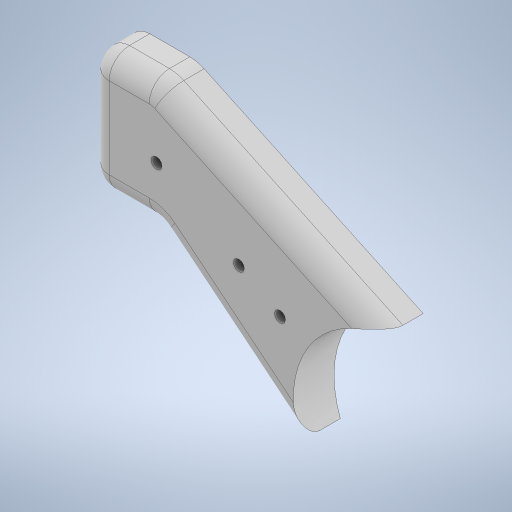
# Autodesk Inventor part: palec2
Saved by Autodesk Inventor 2024.2 (Build 282272000, 272)
## iProperties
Created: 2023-12-27
Part Number: palec2
Material: PLA
Document SubType Name: Modeling
Designer: Konrad
Density: 1 g/cm^3
Appearance: Domyślna
Author: Konrad
Autodesk Inventor part; units mm, degrees
ref_plane "YZ Plane" through (0, 0, 0) normal (1, 0, 0) x (0, 1, 0)
ref_plane "XZ Plane" through (0, 0, 0) normal (0, 1, 0) x (-1, 0, 0)
ref_plane "XY Plane" through (0, 0, 0) normal (0, 0, 1) x (1, 0, 0)
sketch "Szkic1" plane through (0, 0, 0) normal (0, 0, 1) x (1, 0, 0)
  circle A0 centre (0, 0) radius 4
  circle A1 centre (0, 0) radius 12.5 construction
  line L0 (0, 0) -> (-34.641, 20) construction
  line L1 (-44.641, 20) -> (-84.641, 20) construction
  line L2 (-34.641, 20) -> (-34.641, 30) construction
  line L3 (-34.641, 30) -> (5.2954, 11.3229)
  line L4 (-34.641, 20) -> (-34.641, 12) construction
  line L5 (-34.641, 12) -> (-7.8737, -9.7085)
  line L6 (-84.641, 20) -> (-84.641, 30)
  line L7 (-84.641, 30) -> (-34.641, 30)
  line L8 (-34.641, 12) -> (-39.641, 12)
  line L9 (-39.641, 12) -> (-39.641, 15) construction
  line L10 (-39.641, 20) -> (-34.641, 30) construction
  line L11 (-42.641, 20) -> (-37.641, 30) construction
  arc A2 (-1.3611, 14.436) -> (-13.5811, -5.0798) centre (0, 0) ccw
  line L12 (-104.0692, 0) -> (31.9282, 0) construction
  line L13 (-20.4848, 0.5192) -> (-10.0924, 18.5194) construction
  line L14 (-39.641, 12) -> (-44.641, 12)
  line L15 (-44.641, 12) -> (-44.641, 15)
  line L16 (-44.641, 15) -> (-39.641, 15) construction
  arc A3 (-39.641, 15) -> (-44.641, 20) centre (-44.641, 15) ccw
  arc A4 (-39.641, 15) -> (-36.641, 12) centre (-36.641, 15) ccw
  circle A5 centre (-76.641, 25) radius 0.75
  circle A6 centre (-69.641, 25) radius 0.75
  line L17 (-76.641, 25) -> (-69.641, 25) construction
  circle A7 centre (-59.641, 25) radius 0.75
  circle A8 centre (-49.641, 25) radius 0.75
  line L18 (-44.641, 20) -> (-44.641, 30)
  line L19 (-44.641, 15) -> (-44.641, 20)
  circle A9 centre (-16.4545, 9.5) radius 0.8
  circle A10 centre (-22.5167, 13) radius 0.8
  circle A11 centre (-34.641, 20) radius 0.8
  dimension "d0" = 25
  dimension "d1" = 29
  dimension "d2" = 8
  dimension "d4" = 40
  dimension "d5" = 30
  dimension "d6" = 50
  dimension "d7" = 10
  dimension "d8" = 5
  dimension "d9" = 3
  dimension "d10" = 8
  dimension "d11" = 22
  dimension "d16" = 5
  dimension "d17" = 3
  dimension "d20" = 5
  dimension "d21" = 3
  dimension "d23" = 1.5
  dimension "d24" = 1.5
  dimension "d25" = 8
  dimension "d26" = 5
  dimension "d27" = 15
  dimension "d31" = 10
  dimension "d43" = 1.6
  dimension "d45" = 19
  dimension "d46" = 7
  constraints: 38 end point, 16 point on line, 12 centre point, 8 point on circle, 6 perpendicular, 5 horizontal, 4 coincident, 4 tangent, 3 vertical, 2 equal radius, 1 parallel, 4 other
  measures "d0" diameter of A1
  measures "d1" diameter of A2
  measures "d2" diameter of A0
  measures "d4" distance of L0.start L0.end
  measures "d5" angle of L12 L0
  measures "d6" distance of L0.end L1.end
  measures "d7" distance of L1.end L6.end
  measures "d8" distance of L4.end L8.end
  measures "d9" distance of L11.end L2.end
  measures "d10" distance of L8.end L10.start
  measures "d11" distance from line of L0.end L13
  measures "d16" distance of L8.end L14.end
  measures "d17" distance of L14.end L15.end
  measures "d20" radius of A3
  measures "d21" radius of A4
  measures "d23" diameter of A5
  measures "d24" diameter of A6
  measures "d25" distance from line of L6 L17.start
  measures "d26" distance from line of L7 L17.start
  measures "d27" distance from line of L6 L17.end
  measures "d31" distance of L17.end A7.centre
  measures "d43" diameter of A9
  measures "d45" distance of point (0, 0) A9.centre
  measures "d46" distance of A10.centre A9.centre
extrude "Wyciągnięcie proste3" add sketch "Szkic1" along normal blind 6 contours L3 A2 L5 L8 A4 A3 L18 L7 | A3 A4 L8 L14 L15 L19
fillet "Zaokrąglenie4" radius 5 1 edges at (-34.641, 30, 3)
fillet "Zaokrąglenie6" radius 3 2 edges at (-44.641, 12, 3) (-34.641, 12, 3)
fillet "Zaokrąglenie8" radius 3 9 edges at (-34.6675, 29.8809, 6) (-40.1967, 30, 6) (-44.641, 30, 3) (-17.4977, 21.9826, 6) (-43.7623, 12.8787, 6) (-38.6728, 12, 6) (-34.7022, 11.8276, 6) (-23.698, 3.1251, 6) (-44.641, 22.5, 6)
